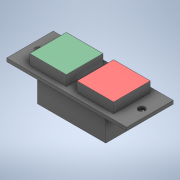
# Autodesk Inventor part: Control-Buttons-Module
Saved by Autodesk Inventor 2022.3 (Build 263350000, 350)
## iProperties
Part Number: Control-Buttons-Module
Material: 一般
Document SubType Name: Modeling
Designer: Masato Kubotera
Density: 1 g/cm^3
Appearance: 滑らか - 黒
Description: CircuitBoard
Mass: 5.19516 g
Surface Area: 35.756 cm^2
Volume: 5.19516 cm^3
Author: Masato Kubotera
Autodesk Inventor part; units mm, degrees
ref_plane "YZ Plane" through (0, 0, 0) normal (1, 0, 0) x (0, 1, 0)
ref_plane "XZ Plane" through (0, 0, 0) normal (0, 1, 0) x (-1, 0, 0)
ref_plane "XY Plane" through (0, 0, 0) normal (0, 0, 1) x (1, 0, 0)
derived "Cockpit_top_frame.ipt"
sketch "スケッチ1" plane through (-75.375, 2.5, -22.5) normal (0, 0, 1) x (1, 0, 0)
  line L0 (-7.825, -1.0151) -> (-7.825, 2.5)
  line L1 (-11.85, 2.5) -> (-8.9, 2.5)
  line L2 (-7.825, 2.5) -> (22.875, 2.5)
  line L3 (22.875, 2.5) -> (22.875, -142.5)
  line L4 (22.875, -70) -> (-12.875, -70) construction
  line L5 (-12.875, -2.5) -> (-12.875, -137.5)
  line L6 (11.639, -0.5602) -> (0, -2.5) construction
  line L7 (0, 0) -> (15, -2.5) construction
  line L8 (13.5651, 0.05) -> (1.4349, 0.05)
  line L9 (-0.05, -1.4349) -> (-0.05, -2.55)
  line L10 (2.05, -2.55) -> (12.95, -2.55)
  line L11 (15.05, -2.55) -> (15.05, -1.4349)
  line L12 (15.05, 0.05) -> (-0.05, -2.55) construction
  line L13 (-0.05, 0.05) -> (15.05, -2.55) construction
  arc A0 (-0.05, -2.55) -> (2.05, -2.55) centre (1, -2.55) ccw
  arc A1 (1.4349, 0.05) -> (-0.05, -1.4349) centre (0.6925, -0.6925) ccw
  line L14 (7.5, -2.55) -> (7.5, 0.05) construction
  arc A2 (12.95, -2.55) -> (15.05, -2.55) centre (14, -2.55) ccw
  arc A3 (15.05, -1.4349) -> (13.5651, 0.05) centre (14.3075, -0.6925) ccw
  circle A4 centre (-3.9375, 0) radius 1.7294 construction
  circle A5 centre (-3.9375, 0) radius 1.6
  line L15 (-7.875, -2.5) -> (-7.875, 2.5)
  line L16 (0, 2.5) -> (15, 2.5)
  line L17 (-13.625, -2.5) -> (-7.875, -2.5)
  line L18 (-12.875, -137.5) -> (-9.3099, -137.5)
  line L19 (-7.825, -138.9849) -> (-7.825, -142.5)
  line L20 (-7.825, -142.5) -> (22.875, -142.5)
  circle A6 centre (-3.9375, -140) radius 1.6
  arc A7 (2.05, -137.45) -> (-0.05, -137.45) centre (1, -137.45) ccw
  line L21 (-0.05, -138.5651) -> (-0.05, -137.45)
  arc A8 (-0.05, -138.5651) -> (1.4349, -140.05) centre (0.6925, -139.3075) ccw
  line L22 (13.5651, -140.05) -> (1.4349, -140.05)
  arc A9 (13.5651, -140.05) -> (15.05, -138.5651) centre (14.3075, -139.3075) ccw
  line L23 (15.05, -137.45) -> (15.05, -138.5651)
  arc A10 (15.05, -137.45) -> (12.95, -137.45) centre (14, -137.45) ccw
  line L24 (2.05, -137.45) -> (12.95, -137.45)
  line L25 (-7.875, -41) -> (14.625, -41)
  line L26 (14.625, -41) -> (14.625, -99)
  line L27 (14.625, -99) -> (-7.875, -99)
  line L28 (-7.875, -99) -> (-7.875, -41)
  line L29 (-7.875, -41) -> (14.625, -99) construction
  line L30 (14.625, -41) -> (-7.875, -99) construction
  line L31 (-5.975, -49.22) -> (12.725, -49.22) construction
  line L32 (12.725, -49.22) -> (12.725, -67.92) construction
  line L33 (12.725, -67.92) -> (-5.975, -67.92) construction
  line L34 (-5.975, -67.92) -> (-5.975, -49.22) construction
  line L35 (-5.975, -49.22) -> (12.725, -67.92) construction
  line L36 (12.725, -49.22) -> (-5.975, -67.92) construction
  line L37 (-4.5608, -48.6342) -> (11.3108, -48.6342) construction
  line L38 (13.3108, -50.6342) -> (13.3108, -66.5058) construction
  line L39 (11.3108, -68.5058) -> (-4.5608, -68.5058) construction
  line L40 (-6.5608, -66.5058) -> (-6.5608, -50.6342) construction
  line L41 (-6.5608, -48.6342) -> (13.3108, -68.5058) construction
  line L42 (13.3108, -48.6342) -> (-6.5608, -68.5058) construction
  arc A11 (-6.5608, -66.5058) -> (-4.5608, -68.5058) centre (-4.5608, -66.5058) ccw construction
  arc A12 (11.3108, -68.5058) -> (13.3108, -66.5058) centre (11.3108, -66.5058) ccw construction
  arc A13 (13.3108, -50.6342) -> (11.3108, -48.6342) centre (11.3108, -50.6342) ccw construction
  arc A14 (-4.5608, -48.6342) -> (-6.5608, -50.6342) centre (-4.5608, -50.6342) ccw construction
  line L43 (12.225, -49.72) -> (-5.475, -49.72)
  line L44 (-5.475, -49.72) -> (-5.475, -67.42)
  line L45 (-5.475, -67.42) -> (12.225, -67.42)
  line L46 (12.225, -67.42) -> (12.225, -49.72)
  line L47 (12.225, -49.72) -> (-5.475, -67.42) construction
  line L48 (-5.475, -49.72) -> (12.225, -67.42) construction
  arc A15 (-4.5608, -71.4942) -> (-6.5608, -73.4942) centre (-4.5608, -73.4942) ccw construction
  line L49 (11.3108, -71.4942) -> (-4.5608, -71.4942) construction
  line L50 (-6.5608, -73.4942) -> (-6.5608, -89.3658) construction
  arc A16 (-6.5608, -89.3658) -> (-4.5608, -91.3658) centre (-4.5608, -89.3658) ccw construction
  line L51 (-4.5608, -91.3658) -> (11.3108, -91.3658) construction
  line L52 (13.3108, -89.3658) -> (13.3108, -73.4942) construction
  arc A17 (13.3108, -73.4942) -> (11.3108, -71.4942) centre (11.3108, -73.4942) ccw construction
  line L53 (-6.5608, -91.3658) -> (3.375, -81.43) construction
  line L54 (13.3108, -91.3658) -> (-6.5608, -71.4942) construction
  arc A18 (11.3108, -91.3658) -> (13.3108, -89.3658) centre (11.3108, -89.3658) ccw construction
  line L55 (3.375, -81.43) -> (13.3108, -71.4942) construction
  circle A19 centre (3.375, -45) radius 2 construction
  circle A20 centre (3.375, -45) radius 1.6
  line L56 (-5.475, -90.28) -> (-5.475, -72.58)
  line L57 (-5.475, -72.58) -> (12.225, -72.58)
  line L58 (12.225, -90.28) -> (-5.475, -90.28)
  line L59 (12.225, -72.58) -> (12.225, -90.28)
  circle A21 centre (3.375, -95) radius 2 construction
  circle A22 centre (3.375, -95) radius 1.6
  line L60 (3.375, -99) -> (3.375, -41) construction
  arc A23 (-9.3099, -2.5) -> (-7.825, -1.0151) centre (-8.5675, -1.7575) ccw
  line L61 (-12.875, -2.5) -> (-9.3099, -2.5)
  arc A24 (-7.825, -138.9849) -> (-9.3099, -137.5) centre (-8.5675, -138.2425) ccw
  line L62 (0.5, 0) -> (14.5, 0)
  line L63 (0, 0) -> (0, -2.5)
  line L64 (0.5, -2.5) -> (14.5, -2.5)
  line L65 (22.875, -110) -> (14.625, -101.75)
  line L66 (14.625, -101.75) -> (14.625, -38.25)
  line L67 (14.625, -38.25) -> (22.875, -30)
  line L68 (12.265, -53.49) -> (-5.515, -53.49)
  line L69 (-5.515, -53.49) -> (-5.515, -86.51)
  line L70 (-5.515, -86.51) -> (12.265, -86.51)
  line L71 (12.265, -86.51) -> (12.265, -53.49)
  line L72 (12.265, -53.49) -> (-5.515, -86.51) construction
  line L73 (-5.515, -53.49) -> (12.265, -86.51) construction
  point P0 (75.375, -2.5)
  point P1 (7.5, -1.25)
  point P2 (22.875, -2.5)
  point P3 (-12.75, -137.5)
  point P4 (3.375, -70)
  point P5 (3.375, -58.57)
  point P6 (3.375, -70)
  point P7 (3.375, -58.57)
  point P8 (-12.875, -2.5)
  point P9 (-12.875, -2.5)
  point P10 (-12.875, -2.5)
  point P11 (-7.825, -2.5)
  point P12 (-12.75, -137.5)
  point P13 (15, -2.5)
  point P14 (12.225, -86.51)
  point P15 (12.225, -53.49)
  point P16 (-5.475, -53.49)
  point P17 (-5.475, -86.51)
  dimension "d5" = 17.78
  dimension "d6" = 33.02
  measures "d5" distance of L70.end L69.end
  measures "d6" distance of L69.end L68.end
extrude "押し出し1" add sketch "スケッチ1" against normal blind 1.6 contours L26 L27 L28 L25 | L46 L68 L44 L43 | L68 L71 L70 L59 L57 L56 L69 L44 L45 L46 | L46 L45 L44 L68 | L70 L56 L57 L59 | L59 L58 L56 L70
extrude "押し出し2" add sketch "スケッチ1" along normal blind 5 contours L46 L68 L44 L43 | L46 L45 L44 L68 | L70 L56 L57 L59 | L59 L58 L56 L70
extrude "Extrusion3" add sketch "スケッチ1" against normal blind 14.1 contours L68 L71 L70 L59 L57 L56 L69 L44 L45 L46 | L46 L45 L44 L68 | L70 L56 L57 L59
